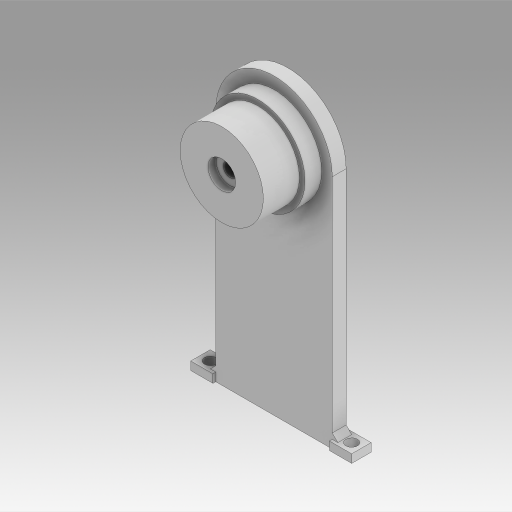
# Autodesk Inventor part: baza_rama_cz2
Saved by Autodesk Inventor 2024.3 (Build 283343000, 343)
## iProperties
Created: 2025-09-01
Part Number: baza_rama_cz2
Material: Ogólny
Document SubType Name: Modeling
Designer: User
Density: 1 g/cm^3
Appearance: Domyślna
Mass: 35.5936 g
Surface Area: 118.638 cm^2
Volume: 35.5936 cm^3
Author: User
Autodesk Inventor part; units mm, degrees
ref_plane "YZ Plane" through (0, 0, 0) normal (1, 0, 0) x (0, 1, 0)
ref_plane "XZ Plane" through (0, 0, 0) normal (0, 1, 0) x (-1, 0, 0)
ref_plane "XY Plane" through (0, 0, 0) normal (0, 0, 1) x (1, 0, 0)
sketch "Szkic1" plane through (0, 0, 0) normal (0, 1, 0) x (-1, 0, 0)
  line L0 (-28.837, -2.0925) -> (29.163, -2.0925)
  line L1 (29.163, 2.9075) -> (29.163, -2.0925)
  line L2 (-28.837, -2.0925) -> (29.163, -2.0925)
  line L3 (29.163, -2.0925) -> (29.163, 2.9075)
  line L4 (29.163, 2.9075) -> (-28.837, 2.9075)
  line L5 (-28.837, 2.9075) -> (-28.837, -2.0925)
  circle A0 centre (-25.337, 0.4075) radius 2.1
  circle A1 centre (-25.337, 0.4075) radius 2.1
  circle A2 centre (25.663, 0.4075) radius 2.1
  circle A3 centre (25.663, 0.4075) radius 2.1
  line L6 (0.163, -2.0925) -> (0.163, 2.9075)
  line L7 (29.163, 0.4075) -> (-28.837, 0.4075)
  line L8 (-20.837, -2.0925) -> (21.163, -2.0925)
  line L9 (21.163, -2.0925) -> (21.163, 2.9075)
  line L10 (21.163, 2.9075) -> (-20.837, 2.9075)
  line L11 (-20.837, 2.9075) -> (-20.837, -2.0925)
  line L12 (-20.837, -2.0925) -> (21.163, 2.9075) construction
  line L13 (21.163, -2.0925) -> (-20.837, 2.9075) construction
  point P0 (0, 0)
  point P1 (0.163, 0.4075)
  dimension "d14" = 42
  dimension "d15" = 5
  dimension "d16" = 4.5
  dimension "d17" = 4.5
  dimension "d18" = 8
  dimension "d19" = 8
  constraints: 28 end point, 7 midpoint, 4 centre point, 4 parallel, 2 coincident, 2 horizontal, 2 perpendicular
  measures "d14" distance of L10.end L9.end
  measures "d15" distance of L9.end L8.end
  measures "d16" distance from line of L11 A0.centre
  measures "d17" distance from line of L9 A2.centre
  measures "d18" distance between parallel lines of L9 L1
  measures "d19" distance between parallel lines of L11 L5
extrude "Wyciągnięcie proste1" add sketch "Szkic1" along normal blind 3 contours L5 L7 A0 L11 L0 | L11 L7 L6 L0 | L5 L4 L11 L7 A0 | L6 L7 L9 L0 | L11 L4 L6 L7 | L9 L7 A2 L1 L0 | L6 L4 L9 L7 | L9 L4 L1 L7 A2
sketch "Szkic2" plane through (0, 3, 0) normal (0, 1, 0) x (1, 0, 0)
  line L0 (-29.163, 2.0925) -> (-29.163, -2.9075) projected
  line L1 (-29.163, -0.4075) -> (-21.163, -0.4075)
  line L2 (28.837, -2.9075) -> (28.837, 2.0925) projected
  line L3 (28.837, -0.4075) -> (20.837, -0.4075)
  line L4 (-29.163, -2.9075) -> (28.837, -2.9075) projected
  line L5 (20.837, -0.4075) -> (-21.163, -0.4075)
  line L6 (-21.163, -0.4075) -> (-21.163, -2.9075)
  line L7 (-21.163, -2.9075) -> (20.837, -2.9075)
  line L8 (20.837, -2.9075) -> (20.837, -0.4075)
  line L9 (28.837, 2.0925) -> (-29.163, 2.0925) projected
  line L10 (-21.163, -0.4075) -> (20.837, -0.4075)
  line L11 (20.837, -0.4075) -> (20.837, 2.0925)
  line L12 (20.837, 2.0925) -> (-21.163, 2.0925)
  line L13 (-21.163, 2.0925) -> (-21.163, -0.4075)
  point P0 (0, 0)
  point P1 (20.837, -2.9075)
  point P2 (20.837, -0.4075)
  dimension "d2" = 8
  dimension "d3" = 8
  constraints: 20 end point, 4 horizontal, 4 parallel, 3 point on line, 2 midpoint, 2 perpendicular
  measures "d2" distance of L1.start L1.end
  measures "d3" distance of L3.start L3.end
extrude "Wyciągnięcie proste2" add sketch "Szkic2" along normal blind 100 contours L9 L11 L5 L13 | L5 L8 L4 L6
fillet "Zaokrąglenie1" radius 21 2 edges at (20.837, 103, 0.4075) (-21.163, 103, 0.4075)
sketch "Szkic3" plane through (-29.163, 0, 2.9075) normal (0, 0, 1) x (1, 0, 0)
  line L0 (29.163, 0) -> (29.163, 81.75)
  circle A0 centre (29.163, 81.75) radius 15
  line L1 (29.163, 0) -> (29.163, 21)
  line L2 (8.163, 0) -> (50.163, 0)
  line L3 (50.163, 0) -> (50.163, 42)
  line L4 (50.163, 42) -> (8.163, 42)
  line L5 (8.163, 42) -> (8.163, 0)
  line L6 (8.163, 0) -> (50.163, 42) construction
  line L7 (50.163, 0) -> (8.163, 42) construction
  dimension "d7" = 81.75
  dimension "d8" = 30
  dimension "d28" = 21
  dimension "d29" = 42
  dimension "d30" = 42
  constraints: 16 end point, 2 midpoint, 2 parallel, 1 centre point, 1 coincident, 1 horizontal, 1 perpendicular, 1 point on line, 1 vertical
  measures "d7" distance of L0.start L0.end
  measures "d8" diameter of A0
  measures "d28" distance of L0.start L1.end
  measures "d29" distance of L4.end L3.end
  measures "d30" distance of L3.end L2.end
extrude "Wyciągnięcie proste3" add sketch "Szkic3" along normal blind 19 contours A0
sketch "Szkic4" plane through (-29.163, 0, 2.9075) normal (0, 0, 1) x (1, 0, 0)
  circle A0 centre (29.163, 81.75) radius 15 projected
  circle A1 centre (29.163, 81.75) radius 17
  point P0 (29.163, 0)
  dimension "d11" = 34
  constraints: 1 centre point, 1 coincident
  measures "d11" diameter of A1
extrude "Wyciągnięcie proste4" add sketch "Szkic4" along normal blind 6
sketch "Szkic5" plane through (0, 0, 0) normal (0, -1, 0) x (1, 0, 0)
  point P0 (0, 0)
sketch "Szkic6" plane through (0, 0, 0) normal (0, -1, 0) x (1, 0, 0)
  line L0 (-21.163, 2.9075) -> (-21.163, -2.0925) projected
  line L1 (-21.163, 2.9075) -> (-29.163, 2.9075)
  line L2 (-29.163, 2.9075) -> (-29.163, -3.0925)
  line L3 (-29.163, -3.0925) -> (-21.163, -3.0925)
  line L4 (-21.163, -3.0925) -> (-21.163, 2.9075)
  line L5 (-21.163, -2.075) -> (-29.163, -2.075)
  line L6 (-29.163, -2.075) -> (-29.163, 3.925)
  line L7 (-29.163, 3.925) -> (-21.163, 3.925)
  line L8 (-21.163, 3.925) -> (-21.163, -2.075)
  line L9 (28.837, -2.0925) -> (-29.163, -2.0925) projected
  line L10 (-29.163, 2.9075) -> (28.837, -2.0925)
  line L11 (28.837, 2.9075) -> (-29.163, -2.0925)
  line L12 (28.837, -2.0925) -> (20.837, -2.0925)
  line L13 (20.837, -2.0925) -> (20.837, 3.9075)
  line L14 (20.837, 3.9075) -> (28.837, 3.9075)
  line L15 (28.837, 3.9075) -> (28.837, -2.0925)
  line L16 (20.837, -2.0925) -> (20.837, 2.9075) projected
  line L17 (20.837, 2.9075) -> (28.837, 2.9075)
  line L18 (28.837, 2.9075) -> (28.837, -3.0925)
  line L19 (28.837, -3.0925) -> (20.837, -3.0925)
  line L20 (20.837, -3.0925) -> (20.837, 2.9075)
  point P0 (0, 0)
  point P1 (20.837, -2.0925)
  point P2 (-21.163, -2.0925)
  dimension "d20" = 6
  dimension "d21" = 6
  dimension "d22" = 6
  constraints: 36 end point, 8 parallel, 4 horizontal, 4 perpendicular, 3 point on line
  measures "d20" distance of L2.end L1.end
  measures "d21" distance of L5.end L6.end
  measures "d22" distance of L12.end L13.end
extrude "Wyciągnięcie proste5" add sketch "Szkic6" against normal blind 3 contours L4 L3 L2 L9 | L9 L18 L19 L20 | L1 L6 L7 L8 | L17 L13 L14 L15
chamfer "Faza1" distance 2 angle 45 2 edges at (20.837, 3, 0.4075) (-21.163, 3, 0.4075)
sketch "Szkic7" plane through (0, 81.75, 21.9075) normal (0, 0, 1) x (1, 0, 0)
  circle A0 centre (0, 0) radius 2.5
  point P0 (0, -81.75)
  dimension "d31" = 5
  constraints: 1 centre point
  measures "d31" diameter of A0
extrude "Wyciągnięcie proste6" cut sketch "Szkic7" against normal blind 53
sketch "Szkic8" plane through (0, 81.75, 21.9075) normal (0, 0, 1) x (1, 0, 0)
  circle A0 centre (0, 0) radius 2.5 projected
  circle A1 centre (0, 0) radius 5
  point P0 (0, -81.75)
  dimension "d34" = 10
  constraints: 1 centre point, 1 coincident
  measures "d34" diameter of A1
extrude "Wyciągnięcie proste7" cut sketch "Szkic8" against normal blind 3
move faces "Przesuń1" translate (0, -3, 0) faces at (28.3703, 3, 0.4075) (22.1703, 3.6667, -0.4258) (6.837, 0, -0.4258) (-0.2091, 29.7561, -2.0925) (-22.4963, 3.6667, 1.2408) (-28.6963, 3, 0.4133)
